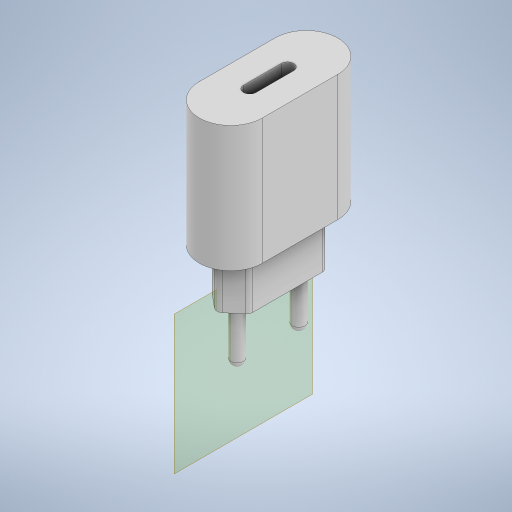
# Autodesk Inventor part: Ctype addapter
Saved by Autodesk Inventor 2024.3 (Build 283343000, 343)
## iProperties
Created: 2024-08-06
Part Number: Ctype addapter
Material: 일반
Document SubType Name: Modeling
Designer: naru4
Density: 1 g/cm^3
Appearance: 기본값
Author: naru4
Autodesk Inventor part; units mm, degrees
ref_plane "YZ Plane" through (0, 0, 0) normal (1, 0, 0) x (0, 1, 0)
ref_plane "XZ Plane" through (0, 0, 0) normal (0, 1, 0) x (-1, 0, 0)
ref_plane "XY Plane" through (0, 0, 0) normal (0, 0, 1) x (1, 0, 0)
sketch "스케치1" plane through (0, 0, 0) normal (0, 1, 0) x (-1, 0, 0)
  arc A0 (5, 6) -> (-5, 6) centre (0, 6) ccw
  arc A1 (-5, -6) -> (5, -6) centre (0, -6) ccw
  line L0 (5, 6) -> (5, -6)
  line L1 (-5, 6) -> (-5, -6)
  point P0 (0, 0)
  constraints: 4 end point, 4 point on circle, 2 centre point, 2 tangent, 1 vertical
extrude "돌출1" add sketch "스케치1" along normal blind 20
sketch "스케치2" plane through (0, 20, 0) normal (0, 1, 0) x (1, 0, 0)
  line L0 (0, 0) -> (0, 3)
  line L1 (0, 3) -> (0, -3)
  circle A0 centre (0, 3) radius 1
  circle A1 centre (0, -3) radius 1
  line L2 (1, 3) -> (1, -3)
  line L3 (-1, -3) -> (-1, 3)
  dimension "d10" = 3
  dimension "d11" = 6
  dimension "d12" = 2
  dimension "d13" = 2
  constraints: 8 end point, 4 point on circle, 2 centre point, 2 coincident, 1 parallel, 1 point on line, 1 tangent, 1 vertical
  measures "d10" distance of L0.start L0.end
  measures "d11" distance of L0.end L1.end
  measures "d12" diameter of A0
  measures "d13" diameter of A1
extrude "돌출2" cut sketch "스케치2" against normal blind 8
sketch "스케치3" plane through (0, 0, 0) normal (0, -1, 0) x (1, 0, 0)
  line L0 (-3, 0) -> (-3, 5.5316)
  line L1 (-2.6402, 6.2998) -> (-0.6402, 7.9665)
  line L2 (-3, 0) -> (-3, -5.5316)
  line L3 (-2.6402, -6.2998) -> (-0.6402, -7.9665)
  line L4 (3, 0) -> (3, 5.5316)
  line L5 (3, 5.5316) -> (3, -5.5316)
  line L6 (2.6402, -6.2998) -> (0.6402, -7.9665)
  line L7 (2.6402, 6.2998) -> (0.6402, 7.9665)
  arc A0 (-0.6402, -7.9665) -> (0.6402, -7.9665) centre (0, -7.1983) ccw
  arc A1 (2.6402, -6.2998) -> (3, -5.5316) centre (2, -5.5316) ccw
  arc A2 (3, 5.5316) -> (2.6402, 6.2998) centre (2, 5.5316) ccw
  arc A3 (0.6402, 7.9665) -> (-0.6402, 7.9665) centre (0, 7.1983) ccw
  arc A4 (-3, -5.5316) -> (-2.6402, -6.2998) centre (-2, -5.5316) ccw
  arc A5 (-2.6402, 6.2998) -> (-3, 5.5316) centre (-2, 5.5316) ccw
  point P0 (0, 0)
  point P1 (-3, -6)
  point P2 (3, -6)
  dimension "d24" = 1
  constraints: 16 end point, 12 point on circle, 12 tangent, 6 centre point, 6 point on line, 5 equal radius
  measures "d24" radius of A0
extrude "돌출3" add sketch "스케치3" along normal blind 8
sketch "스케치4" plane through (0, -8, 0) normal (0, -1, 0) x (1, 0, 0)
  line L0 (0, 0) -> (0, 5)
  line L1 (0, 5) -> (0, -5)
  circle A0 centre (0, 5) radius 1
  circle A1 centre (0, -4.7812) radius 1
  dimension "d27" = 5
  dimension "d28" = 10
  dimension "d29" = 2
  dimension "d30" = 2
  constraints: 4 end point, 2 centre point, 2 point on line, 1 coincident, 1 vertical
  measures "d27" distance of L0.start L0.end
  measures "d28" distance of L0.end L1.end
  measures "d29" diameter of A0
  measures "d30" diameter of A1
extrude "돌출4" add sketch "스케치4" along normal blind 8
ref_plane "작업 평면1" through (0, -16, 4) normal (-1, 0, 0) x (0, 0, 1)
sketch "스케치6" plane through (0, -16, 4) normal (-1, 0, 0) x (0, 0, 1)
  line L0 (0, 0) -> (2, 0) projected
  line L1 (0, -1) -> (1, -1) projected
  arc A0 (0, 0) -> (1, -1) centre (1, 0) ccw
  line L2 (1, -1) -> (1, 0)
  line L3 (1, 0) -> (0, 0)
  point P0 (-4, 16)
  point P1 (1, 0)
  point P2 (1, 0)
  dimension "d35" = 1
  constraints: 4 end point, 2 point on circle, 1 centre point
  measures "d35" radius of A0
revolve "회전1" add sketch "스케치6" angle 360 about axis through (0, -17, 5) along (0, 1, 0)
sketch "스케치7" plane through (0, -16, 4) normal (-1, 0, 0) x (0, 0, 1)
  line L0 (-9.7812, 0) -> (-7.7812, 0) projected
  line L1 (-7.7812, 0) -> (-8.7812, 0)
  line L2 (-8.7812, 0) -> (-8.7812, -1)
  arc A0 (-8.7812, -1) -> (-7.7812, 0) centre (-8.7812, 0) ccw
  point P0 (-4, 16)
  dimension "d37" = 1
  dimension "d38" = 1
  constraints: 4 end point, 2 point on circle, 1 centre point, 1 midpoint, 1 perpendicular
  measures "d37" distance of L1.end L2.end
  measures "d38" radius of A0
revolve "회전2" add sketch "스케치7" angle 360 about axis through (0, -16, -4.7812) along (0, -1, 0)
sketch "스케치8" plane through (0, 12, 0) normal (0, 1, 0) x (1, 0, 0)
  line L0 (0, 0) -> (0, 3)
  line L1 (0, 3) -> (0, -3)
  circle A0 centre (0, -3) radius 0.5
  circle A1 centre (0, 3) radius 0.5
  line L2 (-0.5, -3) -> (-0.5, 3)
  line L3 (0.5, -3) -> (0.5, 3)
  dimension "d40" = 3
  dimension "d41" = 6
  dimension "d42" = 1
  dimension "d43" = 1
  constraints: 8 end point, 4 point on circle, 2 centre point, 2 coincident, 2 tangent, 1 point on line, 1 vertical
  measures "d40" distance of L0.start L0.end
  measures "d41" distance of L0.end L1.end
  measures "d42" diameter of A0
  measures "d43" diameter of A1
extrude "돌출6" add sketch "스케치8" along normal blind 6
